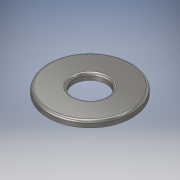
# Autodesk Inventor part: Arruela lisa para 1 quarto
Saved by Autodesk Inventor 2019.4 (Build 234330000, 330)
## iProperties
Created: 2021-04-26
Part Number: Arruela lisa para 1 quarto
Material: Aço, carbono
Document SubType Name: Modeling
Designer: Lattes
Density: 7.85 g/cm^3
Appearance: Semipolido
Author: Lattes
Autodesk Inventor part; units mm, degrees
ref_plane "YZ Plane" through (0, 0, 0) normal (1, 0, 0) x (0, 1, 0)
ref_plane "XZ Plane" through (0, 0, 0) normal (0, 1, 0) x (-1, 0, 0)
ref_plane "XY Plane" through (0, 0, 0) normal (0, 0, 1) x (1, 0, 0)
sketch "Esboço1" plane through (0, 0, 0) normal (0, 1, 0) x (-1, 0, 0)
  circle A0 centre (0, 0) radius 9
  circle A1 centre (0, 0) radius 3.5
  dimension "d0" = 18
  dimension "d1" = 7
  constraints: 2 centre point, 2 coincident
  measures "d0" diameter of A0
  measures "d1" diameter of A1
extrude "Extrusão1" add sketch "Esboço1" along normal blind 1.35
fillet "Arredondamento1" radius 0.5 2 edges at (9, 1.35, 0) (3.5, 1.35, 0)
